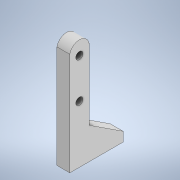
# Autodesk Inventor part: GripperOnS
Saved by Autodesk Inventor 2020 (Build 240168000, 168)
## iProperties
Created: 2020-01-21
Part Number: GripperOnS
Material: Generic
Document SubType Name: Modeling
Designer: tdmp4
Density: 1 g/cm^3
Appearance: Default
Author: tdmp4
Autodesk Inventor part; units mm, degrees
ref_plane "YZ Plane" through (0, 0, 0) normal (1, 0, 0) x (0, 1, 0)
ref_plane "XZ Plane" through (0, 0, 0) normal (0, 1, 0) x (-1, 0, 0)
ref_plane "XY Plane" through (0, 0, 0) normal (0, 0, 1) x (1, 0, 0)
sketch "Sketch1" plane through (0, 0, 0) normal (1, 0, 0) x (0, 1, 0)
  line L0 (0, 0) -> (25.4, 0)
  line L1 (25.4, 0) -> (25.4, -9.525)
  line L2 (25.4, -9.525) -> (0, -9.525)
  line L3 (0, -9.525) -> (0, 0)
  dimension "d0" = 25.4
  dimension "d1" = 9.525
  constraints: 8 end point, 2 parallel, 1 horizontal, 1 perpendicular
  measures "d0" distance of L1.end L2.end
  measures "d1" distance of L2.end L0.start
extrude "Extrusion1" add sketch "Sketch1" along normal blind 6.35
sketch "Sketch2" plane through (6.35, 0, 0) normal (1, 0, 0) x (0, 0, -1)
  line L0 (9.525, 25.4) -> (0, 25.4) projected
  line L1 (0, 0) -> (9.525, 25.4)
  line L2 (9.525, 25.4) -> (0, 25.4)
  line L3 (0, 0) -> (9.525, 0) projected
  line L4 (0, 25.4) -> (9.525, 0)
  circle A0 centre (4.7625, 12.7) radius 9.779
  circle A1 centre (4.7625, 22.479) radius 1.7907
  circle A2 centre (4.7625, 2.921) radius 1.7907
  dimension "d4" = 19.558
  dimension "d5" = 3.5814
  dimension "d6" = 3.5814
  constraints: 6 end point, 3 centre point, 2 point on circle, 1 collinear, 1 midpoint
  measures "d4" diameter of A0
  measures "d5" diameter of A1
  measures "d6" diameter of A2
extrude "Extrusion2" cut sketch "Sketch2" against normal blind 14.2875 contours A1 A0 | A0 A1 | A2 A0 | A0 A2
sketch "Sketch3" plane through (6.35, 0, 0) normal (1, 0, 0) x (0, 0, -1)
  line L0 (9.525, 25.4) -> (0, 25.4) projected
  arc A0 (9.525, 25.4) -> (0, 25.4) centre (4.7625, 24.3714) ccw
  point P0 (0, 0)
  constraints: 2 point on circle, 1 centre point
extrude "Extrusion3" add sketch "Sketch3" against normal blind 6.35
sketch "Sketch4" plane through (6.35, 0, 0) normal (1, 0, 0) x (0, 0, -1)
  line L0 (0, 0) -> (9.525, 0) projected
  line L1 (9.525, 0) -> (0, 0)
  line L2 (0, 0) -> (0, -25.4)
  line L3 (0, -25.4) -> (9.525, -25.4)
  line L4 (9.525, -25.4) -> (9.525, 0)
  dimension "d15" = 25.4
  constraints: 8 end point, 2 parallel, 1 horizontal, 1 perpendicular
  measures "d15" distance of L1.end L2.end
extrude "Extrusion4" add sketch "Sketch4" against normal blind 6.35
sketch "Sketch5" plane through (6.35, 0, 0) normal (1, 0, 0) x (0, 0, -1)
  line L0 (9.525, -25.4) -> (9.525, 25.4) projected
  line L1 (9.525, -9.7563) -> (33.5033, -25.4)
  line L2 (33.5033, -25.4) -> (9.525, -25.4)
  point P0 (0, 0)
  constraints: 4 end point, 1 horizontal, 1 point on line
extrude "Extrusion5" add sketch "Sketch5" against normal blind 6.35
sketch "Sketch6" plane through (6.35, 0, 0) normal (1, 0, 0) x (0, 0, -1)
  line L0 (26.3764, -37.8164) -> (39.194, -37.8164)
  line L1 (39.194, -37.8164) -> (39.194, -17.7508)
  line L2 (39.194, -17.7508) -> (26.3764, -17.7508)
  line L3 (26.3764, -17.7508) -> (26.3764, -37.8164)
  point P0 (0, 0)
  constraints: 8 end point, 2 parallel, 1 horizontal, 1 perpendicular
extrude "Extrusion6" cut sketch "Sketch6" against normal blind 63.5
body "Solid1"
